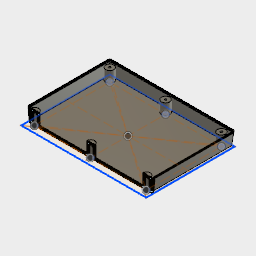
17s-bottom v7 (Autodesk Fusion 360 design; units mm, degrees)
Autodesk Fusion 360 part; units mm, degrees
sketch "Sketch1" plane through (0, 0, 0) normal (0, 1, 0) x (1, 0, 0)
  circle A0 centre (-77.724, 52.324) radius 3.175
  circle A1 centre (0, 52.324) radius 1.397
  circle A2 centre (0, 52.324) radius 3.175
  circle A3 centre (-77.724, 52.324) radius 1.397
  circle A4 centre (-77.724, -52.324) radius 1.397
  line L0 (77.724, -52.324) -> (-77.724, -52.324) construction
  circle A5 centre (0, -52.324) radius 1.397
  circle A6 centre (77.724, 52.324) radius 1.397
  circle A7 centre (77.724, 52.324) radius 3.175
  line L1 (-87.503, 0) -> (87.503, 0) construction
  circle A8 centre (0, -52.324) radius 3.175
  line L2 (87.503, 62.103) -> (87.503, -62.103)
  line L3 (0, 62.103) -> (0, -62.103) construction
  line L4 (-77.724, -52.324) -> (-77.724, 52.324) construction
  circle A9 centre (77.724, -52.324) radius 3.175
  line L5 (-77.724, 52.324) -> (77.724, -52.324) construction
  line L6 (77.724, 52.324) -> (-77.724, -52.324) construction
  circle A10 centre (-77.724, -52.324) radius 3.175
  line L7 (-77.724, 52.324) -> (77.724, 52.324) construction
  line L8 (87.503, -62.103) -> (-87.503, 62.103) construction
  circle A11 centre (77.724, -52.324) radius 1.397
  line L9 (-87.503, -62.103) -> (87.503, 62.103) construction
  line L10 (-87.503, 62.103) -> (87.503, 62.103)
  line L11 (77.724, 52.324) -> (77.724, -52.324) construction
  line L12 (87.503, -62.103) -> (-87.503, -62.103)
  line L13 (-87.503, -62.103) -> (-87.503, 62.103)
  circle A12 centre (77.724, 52.324) radius 4.064
  circle A13 centre (0, 52.324) radius 4.064
  circle A14 centre (-77.724, 52.324) radius 4.064
  circle A15 centre (-77.724, -52.324) radius 4.064
  circle A16 centre (0, -52.324) radius 4.064
  circle A17 centre (77.724, -52.324) radius 4.064
  line L14 (86.36, 60.96) -> (86.36, -60.96)
  line L15 (86.36, -60.96) -> (-86.36, -60.96)
  line L16 (-86.36, -60.96) -> (-86.36, 60.96)
  line L17 (-86.36, 60.96) -> (86.36, 60.96)
  dimension "d1" = 175.006
  dimension "d2" = 124.206
  dimension "d3" = 155.448
  dimension "d4" = 104.648
  dimension "d5" = 6.35
  dimension "d6" = 6.35
  dimension "d7" = 6.35
  dimension "d8" = 6.35
  dimension "d9" = 2.794
  dimension "d10" = 6.35
  dimension "d11" = 2.794
  dimension "d12" = 6.35
  dimension "d13" = 2.794
  dimension "d14" = 2.794
  dimension "d15" = 2.794
  dimension "d35" = 8.128
  dimension "d36" = 8.128
  dimension "d37" = 8.128
  dimension "d38" = 8.128
  dimension "d39" = 8.128
  dimension "d40" = 2.794
  dimension "d41" = 8.128
  dimension "d75" = 1.143
  measures "d1" distance of L8.end L2.start
  measures "d2" distance of L9.start L8.end
  measures "d3" distance of L0.start A4.centre
  measures "d4" distance of L0.start A6.centre
  measures "d5" diameter of A7
  measures "d6" diameter of A0
  measures "d7" diameter of A10
  measures "d8" diameter of A9
  measures "d9" diameter of A6
  measures "d10" diameter of A2
  measures "d11" diameter of A1
  measures "d12" diameter of A8
  measures "d13" diameter of A5
  measures "d14" diameter of A4
  measures "d15" diameter of A3
  measures "d35" diameter of A12
  measures "d36" diameter of A13
  measures "d37" diameter of A14
  measures "d38" diameter of A15
  measures "d39" diameter of A16
  measures "d40" diameter of A11
  measures "d41" diameter of A17
extrude "Extrude1" add sketch "Sketch1" along normal blind 17.78 contours A0 | A1 | A2 | A3 | A4 | A5 | A6 | A7 | A8 | L2 L10 L12 L13 | A9 | A10 | A11 | A12 | A13 | A14 | A15 | A16 | A17 | L14 L15 L16 L17
extrude "Extrude6" add sketch "Sketch1" along normal blind 17.78 contours A0 | A1 | A2 | A3 | A4 | A5 | A6 | A7 | A8 | A9 | A10 | A11 | A12 | A13 | A14 | A15 | A16 | A17
extrude "Extrude7" cut sketch "Sketch1" along normal blind 15.24 contours A0 | A2 | A7 | A8 | A9 | A10
extrude "Extrude8" cut sketch "Sketch1" along normal blind 17.78 contours A1 | A3 | A4 | A5 | A6 | A11
draft "Draft7" angle -5 neutral plane through (0, 17.78, 0) pull (0, 1, 0) 1 faces at (29.1677, 5.9267, 62.103)
draft "Draft8" angle -5 neutral plane through (0, 17.78, 0) pull (0, 1, 0) 1 faces at (-29.1677, 5.9267, -62.103)
draft "Draft9" angle -5 neutral plane through (0, 17.78, 0) pull (0, 1, 0) 1 faces at (-87.503, 11.8533, -20.1825)
draft "Draft10" angle -5 neutral plane through (0, 17.78, 0) pull (0, 1, 0) 1 faces at (87.503, 11.8533, 20.1825)
fillet "Fillet2" radius 2.54 8 edges at (-85.9475, 0, 0) (0, 0, -60.5475) (-86.7252, 8.89, -61.3252) (-86.7252, 8.89, 61.3252) (0, 0, 60.5475) (86.7252, 8.89, 61.3252) (85.9475, 0, 0) (86.7252, 8.89, -61.3252)
shell "Shell2" thickness 2.54 removed faces 1 at (-51.4682, 17.78, -17.0381)
sketch "Sketch3" plane through (0, 17.78, 0) normal (0, 1, 0) x (-1, 0, 0)
  line L0 (84.9533, 59.5533) -> (84.9533, -59.5533)
  line L1 (84.9533, -59.5533) -> (-84.9533, -59.5533)
  line L2 (-84.9533, -59.5533) -> (-84.9533, 59.5533)
  line L3 (-84.9533, 59.5533) -> (84.9533, 59.5533)
  ellipse E0 centre (84.9533, 59.5533) end of major axis (86.763, 61.363) minor radius 2.54 (87.503, 59.5727) -> (84.9727, 62.103) ccw
  line L4 (84.9727, 62.103) -> (-84.9727, 62.103)
  ellipse E1 centre (-84.9533, 59.5533) end of major axis (-86.763, 61.363) minor radius 2.54 (-84.9727, 62.103) -> (-87.503, 59.5727) ccw
  line L5 (-87.503, 59.5727) -> (-87.503, -59.5727)
  ellipse E2 centre (-84.9533, -59.5533) end of major axis (-86.763, -61.363) minor radius 2.54 (-87.503, -59.5727) -> (-84.9727, -62.103) ccw
  line L6 (-84.9727, -62.103) -> (84.9727, -62.103)
  ellipse E3 centre (84.9533, -59.5533) end of major axis (86.763, -61.363) minor radius 2.54 (84.9727, -62.103) -> (87.503, -59.5727) ccw
  line L7 (87.503, -59.5727) -> (87.503, 59.5727)
  line L8 (86.36, -59.5727) -> (86.36, 59.5727)
  spline S0 degree 3 poles (86.36, 59.5727) (86.36, 60.1631) (85.951, 60.7201) (85.3918, 60.8958) (85.257, 60.9382) (85.1151, 60.96) (84.9727, 60.96) knots -0.7816 -0.7816 -0.7816 -0.7816 0.477787 0.477787 0.477787 0.7816 0.7816 0.7816 0.7816
  line L9 (84.9727, 60.96) -> (-84.9727, 60.96)
  spline S1 degree 3 poles (-84.9727, 60.96) (-85.5631, 60.96) (-86.1201, 60.551) (-86.2958, 59.9918) (-86.3382, 59.857) (-86.36, 59.7151) (-86.36, 59.5727) knots -0.7816 -0.7816 -0.7816 -0.7816 0.477787 0.477787 0.477787 0.7816 0.7816 0.7816 0.7816
  line L10 (-86.36, 59.5727) -> (-86.36, -59.5727)
  spline S2 degree 3 poles (-86.36, -59.5727) (-86.36, -60.1631) (-85.951, -60.7201) (-85.3918, -60.8958) (-85.257, -60.9382) (-85.1151, -60.96) (-84.9727, -60.96) knots -0.7816 -0.7816 -0.7816 -0.7816 0.477787 0.477787 0.477787 0.7816 0.7816 0.7816 0.7816
  line L11 (-84.9727, -60.96) -> (84.9727, -60.96)
  spline S3 degree 3 poles (84.9727, -60.96) (85.5631, -60.96) (86.1201, -60.551) (86.2958, -59.9918) (86.3382, -59.857) (86.36, -59.7151) (86.36, -59.5727) knots -0.7816 -0.7816 -0.7816 -0.7816 0.477787 0.477787 0.477787 0.7816 0.7816 0.7816 0.7816
  dimension "d90" = 1.143
extrude "Extrude10" add sketch "Sketch3" along normal blind 1.143 contours E0 L4 E1 L5 E2 L6 E3 L7
ref_plane "WorkPlane2" through (0, 10.16, 51.943) normal (0, 0, -1) x (-1, 0, 0)
